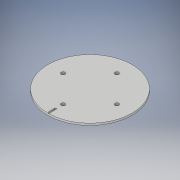
# Autodesk Inventor part: disk_of_zero
Saved by Autodesk Inventor 2019 (Build 230136000, 136)
## iProperties
Created: 2019-12-24
Part Number: disk_of_zero
Material: Типовые
Document SubType Name: Modeling
Designer: Петров Иван
Density: 1 g/cm^3
Appearance: По умолчанию
Author: Петров Иван
Autodesk Inventor part; units mm, degrees
ref_plane "YZ Plane" through (0, 0, 0) normal (1, 0, 0) x (0, 1, 0)
ref_plane "XZ Plane" through (0, 0, 0) normal (0, 1, 0) x (-1, 0, 0)
ref_plane "XY Plane" through (0, 0, 0) normal (0, 0, 1) x (1, 0, 0)
sketch "Эскиз1" plane through (0, 0, 0) normal (0, 1, 0) x (-1, 0, 0)
  circle A0 centre (0, 41.5934) radius 3
  circle A1 centre (41.5934, 0) radius 3
  circle A2 centre (0, -41.5934) radius 3
  arc A3 (-20.609, 31.365) -> (-31.365, 20.609) centre (0, 0) ccw
  arc A4 (-45.7097, 6.2695) -> (-31.365, 20.609) centre (-73.1517, 48.0658) ccw
  arc A5 (-45.7097, 6.2695) -> (-45.7097, -6.2695) centre (-41.5934, 0) ccw
  arc A6 (-31.365, -20.609) -> (-45.7097, -6.2695) centre (-73.1517, -48.0658) ccw
  arc A7 (-31.365, -20.609) -> (-20.609, -31.365) centre (0, 0) ccw
  arc A8 (-6.2695, -45.7097) -> (-20.609, -31.365) centre (-48.0658, -73.1517) ccw
  arc A9 (-6.2695, -45.7097) -> (6.2695, -45.7097) centre (0, -41.5934) ccw
  arc A10 (20.609, -31.365) -> (6.2695, -45.7097) centre (48.0658, -73.1517) ccw
  arc A11 (20.609, -31.365) -> (31.365, -20.609) centre (0, 0) ccw
  arc A12 (45.7097, -6.2695) -> (31.365, -20.609) centre (73.1517, -48.0658) ccw
  arc A13 (45.7097, -6.2695) -> (45.7097, 6.2695) centre (41.5934, 0) ccw
  arc A14 (31.365, 20.609) -> (45.7097, 6.2695) centre (73.1517, 48.0658) ccw
  arc A15 (31.365, 20.609) -> (20.609, 31.365) centre (0, 0) ccw
  arc A16 (6.2695, 45.7097) -> (20.609, 31.365) centre (48.0658, 73.1517) ccw
  arc A17 (6.2695, 45.7097) -> (-6.2695, 45.7097) centre (0, 41.5934) ccw
  arc A18 (-20.609, 31.365) -> (-6.2695, 45.7097) centre (-48.0658, 73.1517) ccw
  circle A19 centre (-41.5934, 0) radius 3
  circle A20 centre (0, 0) radius 65
  dimension "d0" = 130
  constraints: 32 point on circle, 21 centre point, 1 coincident
  measures "d0" diameter of A20
extrude "Выдавливание1" add sketch "Эскиз1" along normal blind 3 contours A18 A17 A16 A15 A14 A13 A12 A11 A10 A9 A8 A7 A6 A5 A4 A3 | A20
sketch "Эскиз2" plane through (0, 3, 0) normal (0, 1, 0) x (1, 0, 0)
  line L0 (0, 0) -> (0, -58.9628)
  line L1 (0, -63.1657) -> (0, -53.2033) construction
  line L2 (1.3029, -63.1657) -> (1.3029, -53.2033)
  line L3 (-1.3029, -53.2033) -> (-1.3029, -63.1657)
  arc A0 (-1.3029, -63.1657) -> (1.3029, -63.1657) centre (0, -63.1657) ccw
  arc A1 (1.3029, -53.2033) -> (-1.3029, -53.2033) centre (0, -53.2033) ccw
  point P0 (0, -58.1845)
  constraints: 10 end point, 4 point on circle, 4 tangent, 2 centre point, 2 point on line, 1 midpoint, 1 parallel, 1 vertical
extrude "Выдавливание2" cut sketch "Эскиз2" against normal blind 3
sketch "Эскиз3" plane through (0, 3, 0) normal (0, 1, 0) x (1, 0, 0)
  arc A0 (1.3029, -53.2033) -> (-1.3029, -53.2033) centre (0, -53.2033) ccw projected
  line L0 (1.3029, -53.2033) -> (1.3029, -63.1657) projected
  arc A1 (-1.3029, -63.1657) -> (1.3029, -63.1657) centre (0, -63.1657) ccw projected
  line L1 (-1.3029, -63.1657) -> (-1.3029, -53.2033) projected
  circle A2 centre (41.5934, 0) radius 3 projected
  circle A3 centre (0, 41.5934) radius 3 projected
  circle A4 centre (-41.5934, 0) radius 3 projected
  circle A5 centre (0, -41.5934) radius 3 projected
  circle A6 centre (0, 0) radius 65 projected
